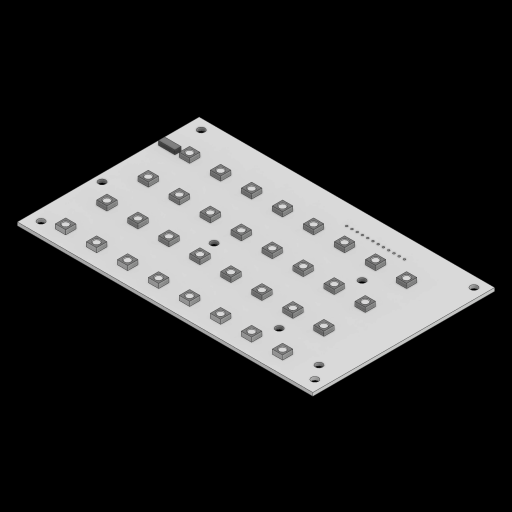
# Autodesk Inventor part: 100_PICO_Mainboard
Saved by Autodesk Inventor 2024 (Build 280153000, 153)
## iProperties
Created: 2023-07-20
Part Number: 100_PICO_Mainboard
Material: Generisch
Document SubType Name: Modeling
Designer: Philipp
Density: 1 g/cm^3
Appearance: Vorgabe
Author: Philipp
Autodesk Inventor part; units mm, degrees
ref_plane "YZ Plane" through (0, 0, 0) normal (1, 0, 0) x (0, 1, 0)
ref_plane "XZ Plane" through (0, 0, 0) normal (0, 1, 0) x (-1, 0, 0)
ref_plane "XY Plane" through (0, 0, 0) normal (0, 0, 1) x (1, 0, 0)
sketch "Skizze1" plane through (0, 0, 0) normal (0, 0, 1) x (1, 0, 0)
  line L0 (0, 0) -> (143, 0)
  line L1 (143, 0) -> (143, 88)
  line L2 (143, 88) -> (0, 88)
  line L3 (0, 88) -> (0, 0)
  dimension "d0" = 143
  dimension "d1" = 88
  constraints: 8 end point, 2 parallel, 1 horizontal, 1 perpendicular
  measures "d0" distance of L2.end L1.end
  measures "d1" distance of L1.end L0.end
extrude "Extrusion1" add sketch "Skizze1" along normal blind 1.6
sketch "Skizze2" plane through (0, 0, 1.6) normal (0, 0, 1) x (1, 0, 0)
  circle A0 centre (6, 83) radius 1.75
  line L0 (0, 0) -> (143, 0) projected
  line L1 (0, 88) -> (0, 0) projected
  circle A1 centre (56.554, 38.657) radius 1.75
  circle A2 centre (3.75, 37.25) radius 1.75
  circle A3 centre (108, 18.725) radius 1.75
  circle A4 centre (138, 6) radius 1.75
  circle A5 centre (133, 13) radius 1.75
  circle A6 centre (108, 58.843) radius 1.75
  circle A7 centre (138, 83) radius 1.75
  circle A8 centre (5.5, 6) radius 1.75
  dimension "d4" = 3.5
  dimension "d5" = 83
  dimension "d6" = 6
  dimension "d7" = 3.5
  dimension "d9" = 3.5
  dimension "d10" = 3.5
  dimension "d11" = 3.5
  dimension "d12" = 3.5
  dimension "d13" = 3.5
  dimension "d14" = 37.25
  dimension "d15" = 38.657
  dimension "d16" = 3.5
  dimension "d17" = 3.75
  dimension "d18" = 3.5
  dimension "d19" = 5.5
  dimension "d20" = 6
  dimension "d21" = 56.554
  dimension "d22" = 58.843
  dimension "d23" = 108
  dimension "d24" = 108
  dimension "d25" = 18.725
  dimension "d26" = 13
  dimension "d27" = 133
  dimension "d28" = 138
  dimension "d29" = 6
  dimension "d30" = 138
  dimension "d31" = 83
  constraints: 9 centre point
  measures "d4" diameter of A0
  measures "d5" distance from line of L0 A0.centre
  measures "d6" distance from line of L1 A0.centre
  measures "d7" diameter of A2
  measures "d9" diameter of A3
  measures "d10" diameter of A4
  measures "d11" diameter of A5
  measures "d12" diameter of A6
  measures "d13" diameter of A7
  measures "d14" distance from line of L0 A2.centre
  measures "d15" distance from line of L0 A1.centre
  measures "d16" diameter of A1
  measures "d17" distance from line of L1 A2.centre
  measures "d18" diameter of A8
  measures "d19" distance from line of L1 A8.centre
  measures "d20" distance from line of L0 A8.centre
  measures "d21" distance from line of L1 A1.centre
  measures "d22" distance from line of L0 A6.centre
  measures "d23" distance from line of L1 A6.centre
  measures "d24" distance from line of L1 A3.centre
  measures "d25" distance from line of L0 A3.centre
  measures "d26" distance from line of L0 A5.centre
  measures "d27" distance from line of L1 A5.centre
  measures "d28" distance from line of L1 A4.centre
  measures "d29" distance from line of L0 A4.centre
  measures "d30" distance from line of L1 A7.centre
  measures "d31" distance from line of L0 A7.centre
extrude "Extrusion2" cut sketch "Skizze2" against normal blind 1.6
sketch "Skizze3" plane through (0, 0, 1.6) normal (0, 0, 1) x (1, 0, 0)
  circle A0 centre (81.4, 78) radius 0.5
  line L0 (0, 0) -> (143, 0) projected
  line L1 (0, 88) -> (0, 0) projected
  dimension "d34" = 1
  dimension "d35" = 78
  dimension "d36" = 81.4
  constraints: 1 centre point
  measures "d34" diameter of A0
  measures "d35" distance from line of L0 A0.centre
  measures "d36" distance from line of A0.centre L1
extrude "Extrusion3" cut sketch "Skizze3" against normal blind 1.6
pattern_linear "Rechteckige Anordnung1" count 12 spacing 2.54 along (1, 0, 0) of "Extrusion3"
sketch "Skizze4" plane through (0, 0, 1.6) normal (0, 0, 1) x (1, 0, 0)
  line L0 (12.125, 11.25) -> (17.125, 11.25)
  line L1 (17.125, 11.25) -> (17.125, 6.25)
  line L2 (17.125, 6.25) -> (12.125, 6.25)
  line L3 (12.125, 6.25) -> (12.125, 11.25)
  line L4 (0, 0) -> (143, 0) projected
  line L5 (0, 88) -> (0, 0) projected
  point P0 (12.125, 8.75)
  point P1 (14.625, 6.25)
  dimension "d42" = 5
  dimension "d43" = 5
  dimension "d44" = 8.75
  dimension "d45" = 14.625
  constraints: 8 end point, 2 midpoint, 2 parallel, 1 horizontal, 1 perpendicular
  measures "d42" distance of L0.start L0.end
  measures "d43" distance of L2.end L0.start
  measures "d44" distance from line of L4 point (12.125, 8.75)
  measures "d45" distance from line of L5 point (14.625, 6.25)
extrude "Extrusion4" add sketch "Skizze4" along normal blind 2.13
sketch "Skizze5" plane through (0, 0, 3.73) normal (0, 0, 1) x (1, 0, 0)
  line L0 (12.125, 6.25) -> (17.125, 6.25) projected
  line L1 (17.125, 6.25) -> (17.125, 11.25) projected
  line L2 (17.125, 11.25) -> (12.125, 11.25) projected
  line L3 (12.125, 11.25) -> (12.125, 6.25) projected
  circle A0 centre (14.625, 8.75) radius 1.8
  point P0 (0, 0)
  dimension "d48" = 3.6
  constraints: 1 centre point
  measures "d48" diameter of A0
extrude "Extrusion5" cut sketch "Skizze5" against normal blind 0.25 contours A0
chamfer "Fasen1" distance 0.25 angle 45 1 edges at (12.825, 8.75, 3.48)
pattern_linear "Rechteckige Anordnung2" count 8 spacing 15 along (1, 0, 0) count 4 spacing 20 along (0, 1, 0) of "Fasen1", "Extrusion5", "Extrusion4"
sketch "Skizze6" plane through (0, 0, 1.6) normal (0, 0, 1) x (1, 0, 0)
  line L0 (2, 69.25) -> (10, 69.25)
  line L1 (10, 69.25) -> (10, 66.25)
  line L2 (10, 66.25) -> (2, 66.25)
  line L3 (2, 66.25) -> (2, 69.25)
  line L4 (12.125, 66.25) -> (17.125, 66.25) projected
  line L5 (12.125, 71.25) -> (12.125, 66.25) projected
  line L6 (0, 88) -> (0, 0) projected
  point P0 (6, 66.25)
  dimension "d60" = 0
  dimension "d61" = 3
  dimension "d62" = 8
  dimension "d64" = 6
  constraints: 8 end point, 2 parallel, 1 horizontal, 1 midpoint, 1 perpendicular
  measures "d60" distance between parallel lines of L4 L2
  measures "d61" distance of L0.end L1.end
  measures "d62" distance of L0.start L0.end
  measures "d64" distance from line of L6 point (6, 66.25)
extrude "Extrusion6" add sketch "Skizze6" along normal blind 2
sketch "Skizze7" plane through (0, 0, 0) normal (0, 0, -1) x (-1, 0, 0)
  line L0 (-135.625, 79.875) -> (-114.625, 79.875)
  line L1 (-114.625, 79.875) -> (-114.625, 28.875)
  line L2 (-114.625, 28.875) -> (-135.625, 28.875)
  line L3 (-135.625, 28.875) -> (-135.625, 79.875)
  line L4 (0, 88) -> (0, 0) projected
  line L5 (0, 0) -> (-143, 0) projected
  point P0 (-125.125, 28.875)
  point P1 (-114.625, 54.375)
  dimension "d67" = 125.125
  dimension "d68" = 54.375
  dimension "d69" = 21
  dimension "d70" = 51
  constraints: 8 end point, 2 midpoint, 2 parallel, 1 horizontal, 1 perpendicular
  measures "d67" distance from line of L4 point (-125.125, 28.875)
  measures "d68" distance from line of L5 point (-114.625, 54.375)
  measures "d69" distance of L0.start L0.end
  measures "d70" distance of L2.end L0.start
extrude "Extrusion7" add sketch "Skizze7" along normal blind 1.6
